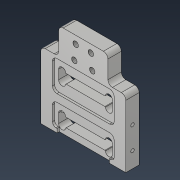
# Autodesk Inventor part: Spulenhalter Hinten
Saved by Autodesk Inventor 2022.1 (Build 261234020, 234B)
## iProperties
Part Number: Spulenhalter Hinten
Material: Aluminium 6061
Document SubType Name: Modeling
Designer: rYan
Density: 2.7 g/cm^3
Appearance: Aluminium - flach
Mass: 16.9891 g
Surface Area: 44.1608 cm^2
Volume: 6.29226 cm^3
Author: rYan
Autodesk Inventor part; units mm, degrees
ref_plane "YZ Plane" through (0, 0, 0) normal (1, 0, 0) x (0, 1, 0)
ref_plane "XZ Plane" through (0, 0, 0) normal (0, 1, 0) x (-1, 0, 0)
ref_plane "XY Plane" through (0, 0, 0) normal (0, 0, 1) x (1, 0, 0)
sketch "Skizze1" plane through (0, 0, 0) normal (0, 1, 0) x (-1, 0, 0)
  line L0 (-19, 0) -> (-19, 42)
  line L1 (-19, 42) -> (19, 42)
  line L2 (19, 42) -> (19, 0)
  line L3 (0, -8.4) -> (0, 50.4) projected
  line L4 (-12.05, 3) -> (-12.05, 7.1)
  line L5 (-8.85, 7.1) -> (8.85, 7.1)
  line L6 (12.05, 7.1) -> (12.05, 3)
  line L7 (8.85, 19.95) -> (-8.85, 19.95)
  line L8 (-12.05, 19.95) -> (-12.05, 24.05)
  line L9 (-8.85, 24.05) -> (8.85, 24.05)
  line L10 (12.05, 24.05) -> (12.05, 19.95)
  line L11 (12.05, 19.95) -> (-12.05, 24.05) construction
  line L12 (-12.05, 19.95) -> (12.05, 24.05) construction
  line L13 (19, 0) -> (-19, 0)
  arc A0 (12.05, 24.05) -> (8.85, 24.05) centre (10.45, 24.05) ccw
  arc A1 (8.85, 19.95) -> (12.05, 19.95) centre (10.45, 19.95) ccw
  arc A2 (-8.85, 24.05) -> (-12.05, 24.05) centre (-10.45, 24.05) ccw
  arc A3 (-12.05, 19.95) -> (-8.85, 19.95) centre (-10.45, 19.95) ccw
  line L14 (12.05, 22) -> (-12.05, 22) construction
  arc A4 (12.05, 7.1) -> (8.85, 7.1) centre (10.45, 7.1) ccw
  arc A5 (-8.85, 7.1) -> (-12.05, 7.1) centre (-10.45, 7.1) ccw
  line L15 (-8.85, 3) -> (8.85, 3)
  arc A6 (8.85, 3) -> (12.05, 3) centre (10.45, 3) ccw
  arc A7 (-12.05, 3) -> (-8.85, 3) centre (-10.45, 3) ccw
  point P0 (0, 0)
  point P1 (0, 22)
  dimension "d0" = 38
  dimension "d1" = 42
  dimension "d4" = 24.1
  dimension "d7" = 4.1
  dimension "d9" = 22
  dimension "d12" = 3.2
  dimension "d13" = 3.2
  dimension "d29" = 3.2
  dimension "d31" = 4.1
  dimension "d32" = 3
  constraints: 30 end point, 16 point on circle, 8 centre point, 7 tangent, 5 midpoint, 5 parallel, 5 point on line, 3 horizontal, 2 collinear, 2 perpendicular, 6 other
  measures "d0" distance of L0.end L1.end
  measures "d1" distance of L0.start L0.end
  measures "d4" distance of L4.end L6.start
  measures "d7" distance of L8.start L8.end
  measures "d9" distance from line of L13 point (0, 22)
  measures "d12" diameter of A0
  measures "d13" diameter of A4
  measures "d29" diameter of A7
  measures "d31" distance between parallel lines of L5 L15
  measures "d32" distance between parallel lines of L15 L13
extrude "Extrusion1" add sketch "Skizze1" along normal mid plane 6 contours L0 L1 L3 L9 A2 L8 A3 L7 L5 A5 L4 A7 L15 L13 | L3 L15 A6 L6 A4 L5 L7 A1 L10 A0 L9 L1 L2 L13
sketch "Skizze2" plane through (0, -3, 0) normal (0, -1, 0) x (1, 0, 0)
  line L0 (-8.85, 24.05) -> (8.85, 24.05) projected
  line L1 (8.85, 19.95) -> (-8.85, 19.95) projected
  line L2 (0, 19.95) -> (0, 24.05) construction
  line L3 (8.85, 24.05) -> (-8.85, 24.05) construction
  line L4 (-11.8, 15.2) -> (11.8, 15.2)
  line L5 (13.8, 17.2) -> (13.8, 26.8)
  line L6 (11.8, 28.8) -> (-11.8, 28.8)
  line L7 (-13.8, 26.8) -> (-13.8, 17.2)
  line L8 (-13.8, 15.2) -> (13.8, 28.8) construction
  line L9 (13.8, 15.2) -> (-13.8, 28.8) construction
  line L10 (13.8, 3.35) -> (13.8, 9.85)
  line L11 (11.8, 11.85) -> (-11.8, 11.85)
  line L12 (-13.8, 9.85) -> (-13.8, 3.35)
  arc A0 (-11.8, 28.8) -> (-13.8, 26.8) centre (-11.8, 26.8) ccw
  arc A1 (-13.8, 17.2) -> (-11.8, 15.2) centre (-11.8, 17.2) ccw
  arc A2 (11.8, 15.2) -> (13.8, 17.2) centre (11.8, 17.2) ccw
  arc A3 (13.8, 26.8) -> (11.8, 28.8) centre (11.8, 26.8) ccw
  arc A4 (-11.8, 11.85) -> (-13.8, 9.85) centre (-11.8, 9.85) ccw
  arc A5 (13.8, 9.85) -> (11.8, 11.85) centre (11.8, 9.85) ccw
  arc A6 (12.2, 1.75) -> (13.8, 3.35) centre (12.2, 3.35) ccw
  arc A7 (-13.8, 3.35) -> (-12.2, 1.75) centre (-12.2, 3.35) ccw
  line L13 (-8.85, 7.1) -> (8.85, 7.1) projected
  line L14 (8.85, 3) -> (-8.85, 3) projected
  line L15 (8.85, 7.1) -> (-8.85, 7.1) construction
  line L16 (0, 7.1) -> (0, 3) construction
  line L17 (-12.2, 1.75) -> (-11.7, 1.75)
  line L18 (-11.7, 1.75) -> (-11.7, 0)
  line L19 (-11.7, 0) -> (11.7, 0)
  line L20 (11.7, 0) -> (11.7, 1.75)
  line L21 (11.7, 1.75) -> (12.2, 1.75)
  line L22 (19, 0) -> (-19, 0) projected
  line L23 (-19, 0) -> (19, 0) projected
  line L24 (-19, 0) -> (19, 0) projected
  point P0 (0, 0)
  point P1 (0, 22)
  point P2 (0, 5.05)
  dimension "d14" = 27.6
  dimension "d15" = 13.6
  dimension "d19" = 2
  dimension "d87" = 1.6
  dimension "d88" = 3.3
  dimension "d89" = 6.8
  dimension "d90" = 11.7
  constraints: 32 end point, 16 point on circle, 15 tangent, 9 point on line, 8 centre point, 8 midpoint, 5 equal radius, 5 perpendicular, 3 horizontal, 3 parallel, 2 collinear, 2 other
  measures "d14" distance of L9.end L8.end
  measures "d15" distance of L8.end L9.start
  measures "d19" radius of A0
  measures "d87" radius of A7
  measures "d88" vertical distance of L17.start point (0, 5.05)
  measures "d89" distance from line of L11 point (0, 5.05)
  measures "d90" distance between parallel lines of L18 L16
extrude "Extrusion2" cut sketch "Skizze2" against normal blind 1
sketch "Skizze3" plane through (0, 0, 0) normal (0, 0, 1) x (1, 0, 0)
  line L0 (-22.4, 0) -> (22.4, 0) projected
  line L1 (0, 22.4) -> (0, -22.4) projected
  point P0 (0, 0)
  point P1 (-16, 0)
  point P2 (16, 0)
  dimension "d20" = 32
  constraints: 2 point on line, 1 symmetric about line
  measures "d20" distance of point (16, 0) point (-16, 0)
hole "Bohrung1" at (-16, 0, 0) at (16, 0, 0) direction (0, 0, 1) diameter 3.242 depth 7 tip angle 118 thread size "M4x0.7" class "6H" standard "ISO Metric profile"
sketch "Skizze5" plane through (0, 3, 0) normal (0, 1, 0) x (1, 0, 0)
  line L0 (0, 8.4) -> (0, -50.4) projected
  point P0 (0, 0)
  point P1 (3.4, -38.5)
  point P2 (-3.4, -38.5)
  point P3 (4, -32)
  point P4 (-4, -32)
  dimension "d41" = 6.8
  dimension "d42" = 38.5
  dimension "d63" = 8
  dimension "d64" = 32
  constraints: 2 symmetric about line
  measures "d41" distance of point (3.4, -38.5) point (-3.4, -38.5)
  measures "d42" vertical distance of point (0, 0) point (-3.4, -38.5)
  measures "d63" distance of point (4, -32) point (-4, -32)
  measures "d64" vertical distance of point (0, 0) point (-4, -32)
hole "Bohrung3" at (3.4, 3, 38.5) at (-3.4, 3, 38.5) at (4, 3, 32) at (-4, 3, 32) direction (0, -1, 0) diameter 2.459 end through all thread size "M3x0.5" class "6H" standard "ANSI Metric M Profile"
sketch "Skizze7" plane through (0, -3, 0) normal (0, -1, 0) x (1, 0, 0)
  arc A0 (-13.8, 17.2) -> (-11.8, 15.2) centre (-11.8, 17.2) ccw projected
  line L0 (-13.8, 17.2) -> (-13.8, 26.8) projected
  arc A1 (-11.8, 28.8) -> (-13.8, 26.8) centre (-11.8, 26.8) ccw projected
  line L1 (-11.8, 28.8) -> (11.8, 28.8) projected
  arc A2 (13.8, 26.8) -> (11.8, 28.8) centre (11.8, 26.8) ccw projected
  line L2 (13.8, 26.8) -> (13.8, 17.2) projected
  arc A3 (11.8, 15.2) -> (13.8, 17.2) centre (11.8, 17.2) ccw projected
  line L3 (11.8, 15.2) -> (-11.8, 15.2) projected
  line L4 (19, 42) -> (-19, 42) projected
  line L5 (-19, 42) -> (-19, 0) projected
  line L6 (11.7, 0) -> (19, 0) projected
  line L7 (-13.8, 3.35) -> (-13.8, 9.85) projected
  arc A4 (-11.8, 11.85) -> (-13.8, 9.85) centre (-11.8, 9.85) ccw projected
  line L8 (-11.8, 11.85) -> (11.8, 11.85) projected
  arc A5 (13.8, 9.85) -> (11.8, 11.85) centre (11.8, 9.85) ccw projected
  line L9 (13.8, 9.85) -> (13.8, 3.35) projected
  line L10 (-19, 0) -> (-11.7, 0) projected
  line L11 (19, 0) -> (19, 42) projected
  line L12 (-19, 0) -> (-19, 42) projected
  line L13 (-19, 42) -> (-11, 42)
  line L14 (-11, 42) -> (-11, 30)
  line L15 (-11, 30) -> (-19, 30)
  line L16 (-19, 30) -> (-19, 42)
  line L17 (19, 42) -> (11, 42)
  line L18 (11, 42) -> (11, 30)
  line L19 (11, 30) -> (19, 30)
  line L20 (19, 30) -> (19, 42)
  line L21 (0, 50.4) -> (0, -8.4) projected
  line L22 (-13.8, 17.2) -> (-13.8, 26.8) construction
  arc A6 (-13.8, 3.35) -> (-12.2, 1.75) centre (-12.2, 3.35) ccw projected
  arc A7 (12.2, 1.75) -> (13.8, 3.35) centre (12.2, 3.35) ccw projected
  line L23 (11.7, 1.75) -> (11.7, 0) projected
  line L24 (-11.7, 0) -> (-11.7, 1.75) projected
  line L25 (-11.7, 1.75) -> (-12.2, 1.75) projected
  line L26 (12.2, 1.75) -> (11.7, 1.75) projected
  point P0 (0, 0)
  dimension "d56" = 12
  dimension "d62" = 22
  constraints: 16 end point, 4 parallel, 2 horizontal, 2 perpendicular, 1 point on line, 2 other
  measures "d56" distance of L17.end L18.end
  measures "d62" distance between parallel lines of L18 L14
extrude "Extrusion4" cut sketch "Skizze7" against normal through all contours L4 L11 L19 L18 | L14 L15 L5 L4
fillet "Rundung1" radius 2 6 edges at (11, 0, 42) (-11, 0, 42) (11, 0, 30) (-11, 0, 30) (-19, 0, 30) (19, 0, 30)
fillet "Rundung2" radius 0.2 10 edges at (8.85, 0.5, 24.05) (-8.85, 0.5, 24.05) (-8.85, 0.5, 19.95) (8.85, 0.5, 19.95) (8.85, 0.5, 7.1) (12.05, 0.5, 3) (-8.85, 0.5, 7.1) (-12.05, 0.5, 3) (-8.85, 0.5, 3) (8.85, 0.5, 3)
sketch "Skizze9" plane through (19, -3, 0) normal (1, 0, 0) x (0, 0, -1)
  line L0 (-50.4, 3) -> (8.4, 3) projected
  line L1 (0, -1.2) -> (0, 7.2) projected
  point P0 (0, 3)
  point P1 (-7, 3)
  point P2 (-17, 3)
  dimension "d77" = 7
  dimension "d78" = 17
  constraints: 2 point on line
  measures "d77" distance from line of point (-7, 3) L1
  measures "d78" distance from line of L1 point (-17, 3)
hole "Bohrung5" at (19, 0, 7) at (19, 0, 17) direction (-1, 0, 0) diameter 1.567 depth 8 tip angle 118 thread size "M2x0.4" class "6H" standard "ISO Metric profile"
mirror "Spiegeln1" about plane through (0, 0, 0) normal (1, 0, 0) of "Bohrung5"
equation "\"d7\" = d10"
equation "\"d13\" = d12"
equation "\"d10\" = 4.1"
